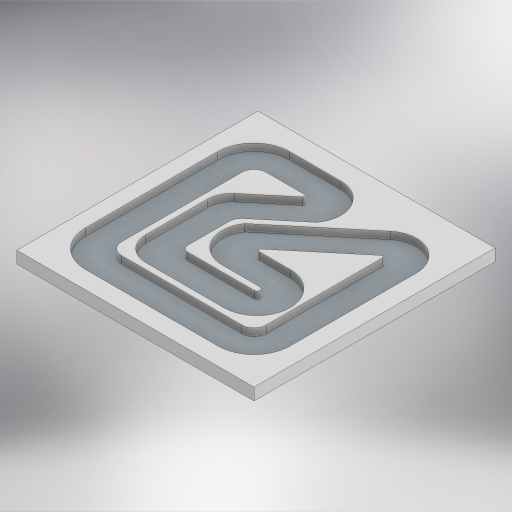
# Autodesk Inventor part: pista
Saved by Autodesk Inventor 2024.2 (Build 282272000, 272)
## iProperties
Created: 2025-02-11
Part Number: pista
Material: Genérico
Document SubType Name: Modeling
Designer: ivani
Density: 38032.1 g/cm^3
Appearance: Valor por defecto
Mass: 1e+13 g
Surface Area: 9.72034e+06 cm^2
Volume: 2.62936e+08 cm^3
Author: ivani
Autodesk Inventor part; units mm, degrees
ref_plane "YZ Plane" through (0, 0, 0) normal (1, 0, 0) x (0, 1, 0)
ref_plane "XZ Plane" through (0, 0, 0) normal (0, 1, 0) x (-1, 0, 0)
ref_plane "XY Plane" through (0, 0, 0) normal (0, 0, 1) x (1, 0, 0)
sketch "Boceto2" plane through (0, 0, 0) normal (0, 1, 0) x (-1, 0, 0)
  line L0 (-3956.5464, 4955.8803) -> (15744.6074, 4955.8803)
  line L1 (15744.6074, 4955.8803) -> (15744.6074, -15071.5867)
  line L2 (15744.6074, -15071.5867) -> (-3956.5464, -15071.5867)
  line L3 (-3956.5464, -15071.5867) -> (-3956.5464, 4955.8803)
  point P0 (0, 0)
  constraints: 8 end point, 2 parallel, 1 horizontal, 1 perpendicular
extrude "Extrusión1" add sketch "Boceto2" against normal blind 1000
sketch "Boceto1" plane through (0, 0, 0) normal (0, 1, 0) x (-1, 0, 0)
  line L0 (0, 0) -> (0, -9679.7438)
  line L1 (1000, 1000) -> (11000, 1000)
  line L2 (12000, 0) -> (12000, -10000)
  arc A0 (12000, 0) -> (11000, 1000) centre (11000, 0) ccw
  arc A1 (1000, 1000) -> (0, 0) centre (1000, 0) ccw
  arc A2 (11000, -11000) -> (12000, -10000) centre (11000, -10000) ccw
  line L3 (500, -10000) -> (6654.0664, -10000) construction
  line L4 (8500, -2000) -> (3000, -2000)
  line L5 (5681.7202, -5265.2332) -> (246.0277, -9794.977)
  line L6 (9000, -2500) -> (9000, -5936.6603)
  line L7 (11000, -11000) -> (7805.5821, -11000)
  line L8 (11500, -1500) -> (11500, -6639.3123)
  line L9 (10780.3688, -8175.7549) -> (7709.5545, -10734.7668)
  line L10 (14500, 500) -> (14500, -10467.1502)
  line L11 (11500, 3500) -> (500, 3500)
  arc A3 (14500, 500) -> (11500, 3500) centre (11500, 500) ccw
  arc A4 (11500, -13467.1502) -> (14500, -10467.1502) centre (11500, -10467.1502) ccw
  arc A5 (500, 3500) -> (-2500, 500) centre (500, 500) ccw
  arc A6 (9000, -2500) -> (8500, -2000) centre (8500, -2500) ccw
  arc A7 (3000, -2000) -> (3000, -2500) centre (3000, -2250) ccw
  arc A8 (5681.7202, -5265.2332) -> (5585.6925, -5000) centre (5585.6925, -5150) ccw
  arc A9 (7709.5545, -10734.7668) -> (7805.5821, -11000) centre (7805.5821, -10850) ccw
  arc A10 (0, -9679.7438) -> (246.0277, -9794.977) centre (150, -9679.7438) ccw
  arc A11 (8196.3535, -6425.0403) -> (6184.5554, -2500) centre (6141.8269, -4999.9992) ccw
  arc A12 (3000, 500) -> (3042.8411, -4999.6663) centre (3000, -2250) ccw
  line L12 (3000, 500) -> (9500, 500)
  line L13 (5585.6925, -5000) -> (3000, -5000)
  arc A13 (5302.3356, -9485.5913) -> (7250, -13467.1502) centre (7250, -11000) ccw
  line L14 (8640.0715, -6704.9756) -> (5302.3356, -9485.5913)
  line L15 (7250, -13467.1502) -> (11500, -13467.1502)
  arc A14 (-2500, -10000) -> (1603.4572, -11918.0524) centre (0, -10000) ccw
  line L16 (1597.0931, -11923.3548) -> (8196.3535, -6425.0403)
  arc A15 (11500, -1500) -> (9500, 500) centre (9500, -1500) ccw
  arc A16 (10780.3688, -8175.7549) -> (11500, -6639.3123) centre (9500, -6639.3123) ccw
  arc A17 (8640.0715, -6704.9756) -> (9000, -5936.6603) centre (8000, -5936.6603) ccw
  line L17 (6184.5554, -2500) -> (3000, -2500)
  line L18 (-2500, -10000) -> (-2500, 500)
  dimension "d0" = 10000
  dimension "d1" = 10000
  dimension "d2" = 10000
  dimension "d21" = 3000
  dimension "d22" = 500
  dimension "d23" = 150
  dimension "d24" = 2000
  dimension "d25" = 2000
  dimension "d26" = 1000
  constraints: 38 end point, 38 point on circle, 21 tangent, 18 centre point, 9 horizontal, 4 equal radius, 4 point on line, 4 vertical, 2 coincident
  measures "d0" distance of L0.start point (0, -10000)
  measures "d1" distance of L1.start L1.end
  measures "d2" distance of L2.start L2.end
  measures "d21" radius of A3
  measures "d22" radius of A6
  measures "d23" radius of A8
  measures "d24" radius of A15
  measures "d25" radius of A16
  measures "d26" radius of A17
extrude "Extrusión2" cut sketch "Boceto1" against normal blind 600 contours L4 A7 L17 A11 L16 A14 L18 A5 L11 A3 L10 A4 L15 A13 L14 A17 L6 A6
